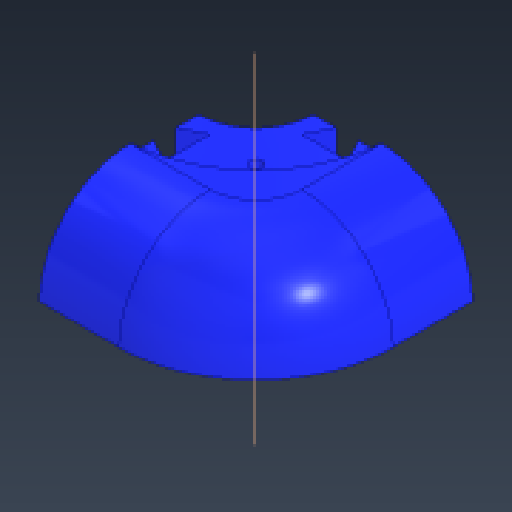
# Autodesk Inventor part: кубик
Saved by Autodesk Inventor 2023.2 (Build 272271030, 271C)
## iProperties
Created: 2025-04-24
Part Number: кубик
Material: Типовые
Document SubType Name: Modeling
Designer: Коноваленко
Density: 1 g/cm^3
Appearance: Синий — малярная краска — глянцевая
Author: Коноваленко
Autodesk Inventor part; units mm, degrees
ref_plane "YZ Plane" through (0, 0, 0) normal (1, 0, 0) x (0, 1, 0)
ref_plane "XZ Plane" through (0, 0, 0) normal (0, 1, 0) x (-1, 0, 0)
ref_plane "XY Plane" through (0, 0, 0) normal (0, 0, 1) x (1, 0, 0)
sketch "Эскиз1" plane through (0, 0, 0) normal (0, 1, 0) x (-1, 0, 0)
  line L0 (47.5, 47.5) -> (-47.5, 47.5)
  line L1 (-47.5, 47.5) -> (-47.5, -18.0259)
  line L2 (22.5, -22.5) -> (47.5, -22.5)
  line L3 (47.5, -22.5) -> (47.5, 47.5)
  line L4 (22.5, -47.5) -> (-47.5, -47.5)
  line L5 (-47.5, -47.5) -> (-47.5, 47.5)
  line L6 (-47.5, 47.5) -> (-7.2151, 47.5)
  line L7 (22.5, -22.5) -> (22.5, -47.5)
  arc A0 (12.5, 47.5) -> (-47.5, -12.5) centre (12.5, -12.5) ccw
  line L8 (47.5, -22.5) -> (47.5, -47.5) construction
  line L9 (47.5, -47.5) -> (22.5, -47.5) construction
  line L10 (-47.5, 47.5) -> (47.5, -47.5) construction
  line L11 (47.5, 47.5) -> (-47.5, -47.5) construction
  point P0 (-12.5, -47.5)
  point P1 (0, 0)
  point P2 (0, 0)
  point P3 (-47.5, -12.5)
  dimension "d21" = 95
  dimension "d22" = 95
  dimension "d23" = 70
  dimension "d24" = 70
  dimension "d45" = 60
  constraints: 24 end point, 4 parallel, 4 perpendicular, 3 point on line, 2 horizontal, 2 midpoint, 2 point on circle, 2 tangent, 1 centre point, 1 coincident, 1 vertical
  measures "d21" distance between parallel lines of L1 L3
  measures "d22" distance from line of point (-12.5, -47.5) L0
  measures "d23" distance between parallel lines of L5 L7
  measures "d24" distance between parallel lines of L2 L0
  measures "d45" radius of A0
extrude "Выдавливание9" add sketch "Эскиз1" along normal mid plane 40
sketch "Эскиз17" plane through (0, 20, 0) normal (0, 1, 0) x (1, 0, 0)
  circle A0 centre (-12.5, 12.5) radius 60
  line L0 (47.5, -47.5) -> (47.5, 47.5) projected
  line L1 (-47.5, -47.5) -> (47.5, -47.5) projected
  point P0 (0, 0)
  point P1 (-12.5, -47.5)
  point P2 (47.5, 12.5)
  dimension "d50" = 120
  constraints: 2 tangent, 1 centre point
  measures "d50" diameter of A0
extrude "Выдавливание17" cut sketch "Эскиз17" against normal up to next contours L0 L1 A0
fillet "Сопряжение4" radius 40 3 edges at (47.5, 20, -30) (-30, 20, 47.5) (29.9264, 20, 29.9264)
sketch "Эскиз13" plane through (0, 20, 0) normal (0, 1, 0) x (1, 0, 0)
  arc A0 (-47.5, -7.5) -> (7.5, 47.5) centre (-52.3071, 52.3071) ccw
  line L0 (7.5, 47.5) -> (-22.5, 47.5) projected
  line L1 (-22.5, 47.5) -> (-22.5, 22.5) projected
  line L2 (-22.5, 22.5) -> (-47.5, 22.5) projected
  line L3 (-47.5, 22.5) -> (-47.5, -7.5) projected
  dimension "d60" = 60
  constraints: 2 point on circle, 1 centre point
  measures "d60" radius of A0
extrude "Выдавливание13" cut sketch "Эскиз13" against normal blind 4
sketch "Эскиз14" plane through (0, 16, 0) normal (0, 1, 0) x (1, 0, 0)
  line L0 (-22.5, 22.5) -> (-22.5, 47.5) projected
  line L1 (7.5, -7.5) -> (-47.5, -7.5) projected
  arc A0 (-47.5, -7.5) -> (7.5, 47.5) centre (-52.3071, 52.3071) ccw projected
  line L2 (-22.5, 22.5) -> (-9.8807, 9.8807) construction
  circle A1 centre (-16.1904, 16.1904) radius 2.6
  point P0 (-47.5, -17.5)
  point P1 (-47.5, -47.5)
  point P2 (47.5, 47.5)
  dimension "d94" = 5.2
  constraints: 2 end point, 1 centre point, 1 midpoint, 1 point on circle
  measures "d94" diameter of A1
extrude "Выдавливание14" cut sketch "Эскиз14" against normal up to surface (36 mm away)
sketch "Эскиз15" plane through (0, 16, 0) normal (0, -1, 0) x (1, 0, 0)
  line L0 (-22.5, -47.5) -> (7.5, -47.5) projected
  line L1 (-2.5, -47.5) -> (2.5, -37.5)
  line L2 (2.5, -37.5) -> (-17.5, -37.5)
  line L3 (-17.5, -37.5) -> (-12.5, -47.5)
  point P0 (0, 0)
  point P1 (17.5, -47.5)
  constraints: 6 end point, 1 horizontal, 8 other
extrude "Выдавливание15" cut sketch "Эскиз15" along normal blind 20
ref_plane "РабПлоскость1" through (-47.5, -20, -47.5) normal (-0.7071068, 0, 0.7071068) x (0, 1, 0)
mirror "Зеркальное отражение1" about plane through (-47.5, -20, -47.5) normal (-0.7071068, 0, 0.7071068) of "Выдавливание15"
sketch "Эскиз19" plane through (-47.5, -20, -22.5) normal (-1, 0, 0) x (0, 0, 1)
  line L0 (60, 0) -> (60, 2.5)
  line L1 (50, 2.5) -> (50, 0)
  line L2 (60, 0) -> (60, -2.5)
  line L3 (60, -2.5) -> (55, -7.5)
  line L4 (55, -7.5) -> (50, -2.5)
  line L5 (50, -2.5) -> (50, 0)
  line L6 (-33, -10) -> (-33, 10)
  line L7 (60, 2.5) -> (50, 2.5)
  line L8 (70, 0) -> (0, 0) projected
  point P0 (22.5, 20)
  point P1 (-33, 0)
  point P2 (40, 0)
  dimension "d68" = 10
  dimension "d69" = 10
  dimension "d70" = 2.5
  dimension "d77" = 20
  dimension "d97" = 90
  dimension "d98" = 135
  dimension "d99" = 83
  dimension "d100" = 2.5
  constraints: 16 end point, 3 parallel, 3 point on line, 2 vertical, 1 midpoint, 1 perpendicular
  measures "d68" distance between parallel lines of L1 L0
  measures "d69" distance from line of L8.start L0
  measures "d70" distance of L0.start L0.end
  measures "d77" distance of L6.start L6.end
  measures "d97" angle of L3 L4
  measures "d98" angle of L3 L2
  measures "d99" distance between parallel lines of L5 L6
  measures "d100" distance of L4.end L1.end
extrude "Выдавливание19" add sketch "Эскиз19" against normal blind 35 separate body
sketch "Эскиз24" plane through (-12.5, -20, -22.5) normal (1, 0, 0) x (0, 0, -1)
  line L0 (-60, 2.5) -> (-60, -2.5) projected
  line L1 (-60, -2.5) -> (-55, -7.5) projected
  line L2 (-55, -7.5) -> (-50, -2.5) projected
  line L3 (-50, -2.5) -> (-50, 2.5) projected
  line L4 (-10, 7.5) -> (-10, -7.5) construction
  line L5 (-50, 2.5) -> (-60, 2.5) projected
  dimension "d89" = 15
  dimension "d101" = 40
  constraints: 2 end point, 1 vertical
  measures "d89" distance of L4.start L4.end
  measures "d101" distance between parallel lines of L3 L4
mirror "Зеркальное отражение3" about plane through (-47.5, -20, -47.5) normal (-0.7071068, 0, 0.7071068) of "Выдавливание19" bodies 2
revolve "Вращение5" add sketch "Эскиз24" angle 90 about axis through (-12.5, -12.5, -12.5) along (0, 1, 0) bodies 2
combine bodies "Комбинировать4" operation type subtract main body 1 bodies to subtract 2 keep tools yes
chamfer "Фаска2" distance 2 angle 45 4 edges at (-47.5, -25, 30) (-47.5, -25, 35) (30, -25, -47.5) (35, -25, -47.5)
fillet "Сопряжение5" radius 25 1 edges at (-22.5, -2, -22.5)
